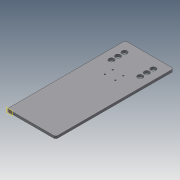
# Autodesk Inventor part: Z-table
Saved by Autodesk Inventor 2014 SP1 (Build 180222100, 222)
## iProperties
Created: 2014-04-10
Part Number: Z-table
Material: Generic
Document SubType Name: Modeling
Designer: tom
Density: 1 g/cm^3
Appearance: Default
Author: tom
Autodesk Inventor part; units mm, degrees
ref_plane "YZ Plane" through (0, 0, 0) normal (1, 0, 0) x (0, 1, 0)
ref_plane "XZ Plane" through (0, 0, 0) normal (0, 1, 0) x (-1, 0, 0)
ref_plane "XY Plane" through (0, 0, 0) normal (0, 0, 1) x (1, 0, 0)
ref_plane "Work Plane1" through (33.3916, -139.4155, 142.8527) normal (0, 0, 1) x (1, 0, 0)
sketch "Sketch1" plane through (33.3916, -139.4155, 142.8527) normal (0, 0, 1) x (1, 0, 0)
  line L0 (-4.0384, 3.4) -> (113.4116, 3.4)
  line L1 (54.6866, 21.1837) -> (54.6866, -18.7057) construction
  line L2 (-4.0384, 3.4) -> (-4.0384, -2.26)
  line L3 (-4.0384, -2.26) -> (113.4116, -2.26)
  line L4 (113.4116, -2.26) -> (113.4116, 3.4)
  dimension "d0" = 5.66
  constraints: 10 end point, 3 perpendicular, 1 parallel
  measures "d0" distance of L0.start L2.end
extrude "Extrusion1" add sketch "Sketch1" against normal blind 286.324
sketch "Sketch2" plane through (29.3531, -141.6755, 142.8527) normal (0, -1, 0) x (1, 0, 0)
  line L0 (117.45, 0) -> (0, 0) projected
  line L1 (117.45, -286.324) -> (0, -286.324) projected
  line L2 (58.725, 0) -> (58.725, -286.324) construction
  line L3 (46.025, -191.074) -> (71.425, -191.074) construction
  line L4 (71.425, -191.074) -> (71.425, -210.124) construction
  line L5 (71.425, -210.124) -> (46.025, -210.124) construction
  line L6 (46.025, -210.124) -> (46.025, -191.074) construction
  circle A0 centre (46.025, -191.074) radius 1.5875
  circle A1 centre (71.425, -191.074) radius 1.5875
  circle A2 centre (71.425, -210.124) radius 1.5875
  circle A3 centre (46.025, -210.124) radius 1.5875
  circle A4 centre (23.8, -260.924) radius 6.35
  circle A5 centre (23.8, -245.049) radius 6.35
  circle A6 centre (23.8, -229.174) radius 6.35
  circle A7 centre (93.65, -260.924) radius 6.35
  circle A8 centre (93.65, -245.049) radius 6.35
  circle A9 centre (93.65, -229.174) radius 6.35
  point P0 (-29.3531, -142.8527)
  dimension "d4" = 25.4
  dimension "d5" = 19.05
  dimension "d6" = 76.2
  dimension "d7" = 12.7
  dimension "d8" = 3.175
  dimension "d9" = 3.175
  dimension "d10" = 3.175
  dimension "d11" = 3.175
  dimension "d12" = 12.7
  dimension "d13" = 12.7
  dimension "d14" = 15.875
  dimension "d15" = 25.4
  dimension "d16" = 12.7
  dimension "d17" = 15.875
  dimension "d18" = 12.7
  dimension "d19" = 12.7
  dimension "d20" = 12.7
  dimension "d21" = 15.875
  dimension "d22" = 15.875
  dimension "d23" = 25.4
  dimension "d24" = 34.925
  dimension "d25" = 34.925
  constraints: 10 centre point, 10 end point, 4 coincident, 2 midpoint, 2 parallel, 1 horizontal, 1 perpendicular
  measures "d4" distance of L4.end L5.end
  measures "d5" distance of L3.end L4.end
  measures "d6" distance from line of L1 L5.end
  measures "d7" distance from line of L2 L5.end
  measures "d8" diameter of A0
  measures "d9" diameter of A1
  measures "d10" diameter of A2
  measures "d11" diameter of A3
  measures "d12" diameter of A4
  measures "d13" diameter of A5
  measures "d14" distance of A4.centre A5.centre
  measures "d15" distance from line of L1 A4.centre
  measures "d16" diameter of A6
  measures "d17" distance of A5.centre A6.centre
  measures "d18" diameter of A7
  measures "d19" diameter of A8
  measures "d20" diameter of A9
  measures "d21" distance of A8.centre A7.centre
  measures "d22" distance of A9.centre A8.centre
  measures "d23" distance from line of L1 A7.centre
  measures "d24" distance from line of L2 A4.centre
  measures "d25" distance from line of L2 A7.centre
extrude "Extrusion2" cut sketch "Sketch2" against normal blind 5.66
chamfer "Chamfer1" distance 3.175 angle 45 4 edges at (146.8031, -138.8455, 142.8527) (29.3531, -138.8455, 142.8527) (29.3531, -138.8455, -143.4713) (146.8031, -138.8455, -143.4713)
body "Solid1"
